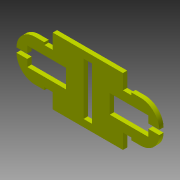
# Autodesk Inventor part: Lock2
Saved by Autodesk Inventor 2014 (Build 180170000, 170)
## iProperties
Created: 2014-11-24
Part Number: Lock2
Material: Generic
Document SubType Name: Modeling
Designer: JLM
Density: 1 g/cm^3
Appearance: Default
Author: JLM
Autodesk Inventor part; units mm, degrees
ref_plane "YZ Plane" through (0, 0, 0) normal (1, 0, 0) x (0, 1, 0)
ref_plane "XZ Plane" through (0, 0, 0) normal (0, 1, 0) x (-1, 0, 0)
ref_plane "XY Plane" through (0, 0, 0) normal (0, 0, 1) x (1, 0, 0)
sketch "Sketch1" plane through (0, 0, 0) normal (0, 0, 1) x (1, 0, 0)
  line L0 (48.6537, 0) -> (48.6537, 14.1161)
  line L1 (48.6537, 14.1161) -> (29.6037, 14.1161)
  line L2 (29.6037, 14.1161) -> (29.6037, 12.446)
  line L3 (29.6037, 12.446) -> (23.8887, 12.446)
  line L4 (12.2521, 0) -> (48.6537, 0)
  line L5 (23.8887, 12.446) -> (23.8887, 22.6695)
  line L6 (23.8887, 22.6695) -> (0, 22.6695)
  line L7 (0, 0) -> (2.921, 0)
  line L8 (2.921, 0) -> (2.921, 17.78)
  line L9 (2.921, 17.78) -> (0, 17.78)
  line L10 (0, 17.78) -> (0, 0)
  line L11 (14.9304, 6.35) -> (14.9304, 0)
  line L12 (48.6537, 1.5875) -> (41.275, 1.5875)
  line L13 (41.275, 1.5875) -> (41.275, 6.35)
  line L14 (41.275, 6.35) -> (14.9304, 6.35)
  line L15 (48.6537, 0) -> (48.6537, -14.116)
  line L16 (48.6537, -14.116) -> (29.6037, -14.116)
  line L17 (29.6037, -14.116) -> (29.6037, -12.446)
  line L18 (29.6037, -12.446) -> (23.8887, -12.446)
  line L19 (23.8887, -12.446) -> (23.8887, -22.6695)
  line L20 (23.8887, -22.6695) -> (0, -22.6695)
  line L21 (2.921, 0) -> (2.921, -17.78)
  line L22 (2.921, -17.78) -> (0, -17.78)
  line L23 (0, -17.78) -> (0, 0)
  line L24 (14.9304, -6.35) -> (14.9304, 0)
  line L25 (48.6537, -1.5875) -> (41.275, -1.5875)
  line L26 (41.275, -1.5875) -> (41.275, -6.35)
  line L27 (41.275, -6.35) -> (14.9304, -6.35)
  line L28 (-48.6537, 0) -> (-48.6537, 14.1161)
  line L29 (-48.6537, 14.1161) -> (-29.6037, 14.1161)
  line L30 (-29.6037, 14.1161) -> (-29.6037, 12.446)
  line L31 (-29.6037, 12.446) -> (-23.8887, 12.446)
  line L32 (-12.2521, 0) -> (-48.6537, 0)
  line L33 (-23.8887, 12.446) -> (-23.8887, 22.6695)
  line L34 (-23.8887, 22.6695) -> (0, 22.6695)
  line L35 (0, 0) -> (-2.921, 0)
  line L36 (-2.921, 0) -> (-2.921, 17.78)
  line L37 (-2.921, 17.78) -> (0, 17.78)
  line L38 (-14.9304, 6.35) -> (-14.9304, 0)
  line L39 (-48.6537, 1.5875) -> (-41.275, 1.5875)
  line L40 (-41.275, 1.5875) -> (-41.275, 6.35)
  line L41 (-41.275, 6.35) -> (-14.9304, 6.35)
  line L42 (-14.9304, -6.35) -> (-14.9304, 0)
  line L43 (-23.8887, -12.446) -> (-23.8887, -22.6695)
  line L44 (-23.8887, -22.6695) -> (0, -22.6695)
  line L45 (-2.921, 0) -> (-2.921, -17.78)
  line L46 (-2.921, -17.78) -> (0, -17.78)
  line L47 (-29.6037, -12.446) -> (-23.8887, -12.446)
  line L48 (-29.6037, -14.116) -> (-29.6037, -12.446)
  line L49 (-41.275, -6.35) -> (-14.9304, -6.35)
  line L50 (-41.275, -1.5875) -> (-41.275, -6.35)
  line L51 (-48.6537, -14.116) -> (-29.6037, -14.116)
  line L52 (-48.6537, -1.5875) -> (-41.275, -1.5875)
  line L53 (-48.6537, 0) -> (-48.6537, -14.116)
  dimension "d0" = 14.116
  dimension "d1" = 19.05
  dimension "d6" = 12.446
  dimension "d7" = 22.6695
  dimension "d8" = 23.8887
  dimension "d9" = 5.715
  dimension "d10" = 2.921
  dimension "d11" = 17.78
  constraints: 108 end point, 36 symmetric about line, 8 perpendicular, 8 point on line, 4 parallel, 1 horizontal
  measures "d0" distance of L0.start L0.end
  measures "d1" distance of L0.end L1.end
  measures "d6" distance between parallel lines of L4 L3
  measures "d7" distance between parallel lines of L4 L6
  measures "d8" distance from line of L5 L7.start
  measures "d9" distance of L2.end L3.end
  measures "d10" distance of L9.end L8.end
  measures "d11" distance of L8.end L7.end
extrude "Extrusion1" add sketch "Sketch1" along normal blind 2.921 contours L12 L13 L14 L11 L24 L27 L26 L25 L15 L16 L17 L18 L19 L20 L44 L43 L47 L48 L51 L53 L52 L50 L49 L42 L38 L41 L40 L39 L28 L29 L30 L31 L33 L34 L6 L5 L3 L2 L1 L0
fillet "Fillet1" radius 12.7 4 edges at (48.6537, 14.1161, 1.4605) (48.6537, -14.116, 1.4605) (-48.6537, -14.116, 1.4605) (-48.6537, 14.1161, 1.4605)
body "Solid1"
